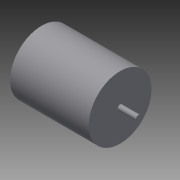
# Autodesk Inventor part: motor
Saved by Autodesk Inventor 2014 (Build 180170000, 170)
## iProperties
Created: 2013-05-23
Part Number: motor
Material: Generisch
Document SubType Name: Modeling
Designer: hartmann
Density: 1 g/cm^3
Appearance: Vorgabe
Author: hartmann
Autodesk Inventor part; units mm, degrees
ref_plane "YZ Plane" through (0, 0, 0) normal (1, 0, 0) x (0, 1, 0)
ref_plane "XZ Plane" through (0, 0, 0) normal (0, 1, 0) x (-1, 0, 0)
ref_plane "XY Plane" through (0, 0, 0) normal (0, 0, 1) x (1, 0, 0)
sketch "Skizze1" plane through (0, 0, 0) normal (1, 0, 0) x (0, 1, 0)
  circle A0 centre (0, 0) radius 12
  line L0 (-7.8852, 9.0456) -> (7.8852, 9.0456)
  line L1 (-7.8852, -9.0456) -> (7.8852, -9.0456)
  dimension "d0" = 24
  constraints: 4 end point, 4 point on circle, 2 parallel, 1 centre point, 1 coincident, 1 horizontal
  measures "d0" diameter of A0
extrude "Extrusion1" add sketch "Skizze1" along normal blind 30
sketch "Skizze2" plane through (30, 0, 0) normal (1, 0, 0) x (0, 0, -1)
  circle A0 centre (0, 0) radius 12 projected
  circle A1 centre (0, 0) radius 1
  dimension "d3" = 2
  constraints: 1 centre point, 1 coincident
  measures "d3" diameter of A1
extrude "Extrusion2" add sketch "Skizze2" along normal blind 7 contours A1
